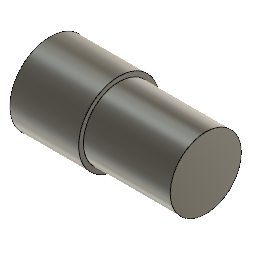
moters v1 (Autodesk Fusion 360 design; units mm, degrees)
Autodesk Fusion 360 part; units mm, degrees
sketch "Sketch1" plane through (0, 0, 0) normal (1, 0, 0) x (0, 0, -1)
  circle A0 centre (-86.36, 0) radius 13.589
  dimension "d92" = 27.178
  dimension "d98" = 0
  dimension "d99" = 0
  dimension "d100" = 0
  dimension "d101" = 0
  measures "d92" diameter of A0
extrude "Extrude1" add sketch "Sketch1" along normal blind 23.2156
sketch "Sketch2" plane through (23.2156, 0, 0) normal (1, 0, 0) x (0, 0, -1)
  circle A0 centre (-86.36, 0) radius 13.589
  circle A1 centre (-86.36, 0) radius 11.9888
  dimension "d95" = 23.9776
  measures "d95" diameter of A1
extrude "Extrude2" add sketch "Sketch2" along normal blind 29.2354 contours A1
